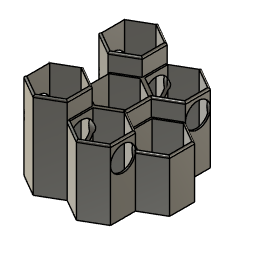
hexagone_rangement v3 (Autodesk Fusion 360 design; units mm, degrees)
Autodesk Fusion 360 part; units mm, degrees
sketch "Esquisse1" plane through (0, 0, 0) normal (0, 0, 1) x (1, 0, 0)
  line L0 (12.5, 7.2169) -> (0, 14.4338)
  line L1 (0, 14.4338) -> (-12.5, 7.2169)
  line L2 (-12.5, 7.2169) -> (-12.5, -7.2169)
  line L3 (-12.5, -7.2169) -> (0, -14.4338)
  line L4 (0, -14.4338) -> (12.5, -7.2169)
  line L5 (12.5, -7.2169) -> (12.5, 7.2169)
  line L6 (0, 14.4338) -> (12.5, 7.2169)
  line L7 (12.5, 7.2169) -> (25, 14.4338)
  line L8 (25, 14.4338) -> (25, 28.8675)
  line L9 (25, 28.8675) -> (12.5, 36.0844)
  line L10 (12.5, 36.0844) -> (0, 28.8675)
  line L11 (0, 28.8675) -> (0, 14.4338)
  line L12 (0, 28.8675) -> (12.5, 36.0844)
  line L13 (12.5, 36.0844) -> (12.5, 50.5181)
  line L14 (12.5, 50.5181) -> (0, 57.735)
  line L15 (0, 57.735) -> (-12.5, 50.5181)
  line L16 (-12.5, 50.5181) -> (-12.5, 36.0844)
  line L17 (-12.5, 36.0844) -> (0, 28.8675)
  line L18 (12.5, 7.2169) -> (12.5, -7.2169)
  line L19 (12.5, -7.2169) -> (25, -14.4338)
  line L20 (25, -14.4338) -> (37.5, -7.2169)
  line L21 (37.5, -7.2169) -> (37.5, 7.2169)
  line L22 (37.5, 7.2169) -> (25, 14.4338)
  line L23 (25, 14.4338) -> (12.5, 7.2169)
  line L24 (12.5, 36.0844) -> (25, 28.8675)
  line L25 (25, 28.8675) -> (37.5, 36.0844)
  line L26 (37.5, 36.0844) -> (37.5, 50.5181)
  line L27 (37.5, 50.5181) -> (25, 57.735)
  line L28 (25, 57.735) -> (12.5, 50.5181)
  line L29 (12.5, 50.5181) -> (12.5, 36.0844)
  line L30 (25, 28.8675) -> (25, 14.4338)
  line L31 (25, 14.4338) -> (37.5, 7.2169)
  line L32 (37.5, 7.2169) -> (50, 14.4338)
  line L33 (50, 14.4338) -> (50, 28.8675)
  line L34 (50, 28.8675) -> (37.5, 36.0844)
  line L35 (37.5, 36.0844) -> (25, 28.8675)
  line L36 (0, 13.2791) -> (-11.5, 6.6395)
  line L37 (-11.5, 6.6395) -> (-11.5, -6.6395)
  line L38 (-11.5, -6.6395) -> (0, -13.2791)
  line L39 (0, -13.2791) -> (11.5, -6.6395)
  line L40 (11.5, -6.6395) -> (11.5, 6.6395)
  line L41 (0, 13.2791) -> (11.5, 6.6395)
  line L42 (13.5, -6.6395) -> (25, -13.2791)
  line L43 (25, -13.2791) -> (36.5, -6.6395)
  line L44 (36.5, -6.6395) -> (36.5, 6.6395)
  line L45 (36.5, 6.6395) -> (25, 13.2791)
  line L46 (25, 13.2791) -> (13.5, 6.6395)
  line L47 (13.5, -6.6395) -> (13.5, 6.6395)
  line L48 (26, 15.0111) -> (26, 28.2902)
  line L49 (26, 28.2902) -> (37.5, 34.9297)
  line L50 (49, 28.2902) -> (37.5, 34.9297)
  line L51 (49, 15.0111) -> (49, 28.2902)
  line L52 (37.5, 8.3716) -> (49, 15.0111)
  line L53 (37.5, 8.3716) -> (26, 15.0111)
  line L54 (1, 28.2902) -> (12.5, 34.9297)
  line L55 (24, 28.2902) -> (12.5, 34.9297)
  line L56 (24, 28.2902) -> (24, 15.0111)
  line L57 (12.5, 8.3716) -> (24, 15.0111)
  line L58 (12.5, 8.3716) -> (1, 15.0111)
  line L59 (1, 28.2902) -> (1, 15.0111)
  line L60 (13.5, 36.6617) -> (13.5, 49.9408)
  line L61 (25, 56.5803) -> (13.5, 49.9408)
  line L62 (36.5, 49.9408) -> (25, 56.5803)
  line L63 (36.5, 36.6617) -> (36.5, 49.9408)
  line L64 (36.5, 36.6617) -> (25, 30.0222)
  line L65 (25, 30.0222) -> (13.5, 36.6617)
  line L66 (11.5, 36.6617) -> (11.5, 49.9408)
  line L67 (11.5, 49.9408) -> (0, 56.5803)
  line L68 (0, 56.5803) -> (-11.5, 49.9408)
  line L69 (-11.5, 49.9408) -> (-11.5, 36.6617)
  line L70 (-11.5, 36.6617) -> (0, 30.0222)
  line L71 (0, 30.0222) -> (11.5, 36.6617)
  point P0 (12.5, 21.6506)
  point P1 (0, 43.3013)
  point P2 (25, 0)
  point P3 (25, 43.3013)
  point P4 (37.5, 21.6506)
  dimension "d5" = 25
  dimension "d10" = 1
  dimension "d11" = 1
  measures "d5" distance of L2 L5
extrude "Extrusion1" add sketch "Esquisse1" along normal blind 50 contours L0 L1 L2 L3 L4 L5 L6 L18 | L10 L12 L13 L14 L15 L16 L17 L29 makes body 1 at (12.5, -2.4056, 16.6667) makes body 2 at (-4.1667, 55.3294, 16.6667)
extrude "Extrusion2" add sketch "Esquisse1" along normal blind 40 contours L5 L7 L18 L19 L20 L21 L22 L23 L31 | L0 L6 L7 L8 L9 L10 L11 L12 L23 L24 L30 | L9 L13 L24 L25 L26 L27 L28 L29 L35 bodies 1 2
extrude "Extrusion3" add sketch "Esquisse1" along normal blind 30 contours L8 L22 L25 L30 L31 L32 L33 L34 L35 bodies 1
extrude "Extrusion4" add sketch "Esquisse1" along normal blind 2 contours L36 L37 L38 L39 L40 L41 | L42 L43 L44 L45 L46 L47 | L48 L49 L50 L51 L52 L53 | L54 L55 L56 L57 L58 L59 | L60 L61 L62 L63 L64 L65 | L66 L67 L68 L69 L70 L71 bodies 1
sketch "Esquisse3" plane through (37.5, 0, 0) normal (1, 0, 0) x (0, 1, 0)
  line L0 (-7.2169, 0) -> (7.2169, 0)
  line L1 (7.2169, 0) -> (7.2169, 30)
  line L2 (7.2169, 30) -> (7.2169, 40)
  line L3 (7.2169, 40) -> (-7.2169, 40)
  line L4 (-7.2169, 40) -> (-7.2169, 0)
  circle A0 centre (0, 30) radius 7.2169
  constraint coincident L1.end A0
extrude "Extrusion5" cut sketch "Esquisse3" against normal blind 71 contours A0 bodies 1
sketch "Esquisse4" plane through (37.5, 0, 0) normal (1, 0, 0) x (0, 1, 0)
  line L0 (36.0844, 0) -> (50.5181, 0)
  line L1 (50.5181, 0) -> (50.5181, 40)
  line L2 (50.5181, 40) -> (36.0844, 40)
  line L3 (36.0844, 40) -> (36.0844, 30)
  line L4 (36.0844, 30) -> (36.0844, 0)
  circle A0 centre (43.3013, 30) radius 7.2169
extrude "Extrusion6" cut sketch "Esquisse4" against normal blind 55 contours A0 bodies 1
fillet "Congé1" radius 1 3 edges at (43.75, 10.8253, 30) (50, 21.6506, 30) (43.75, 32.476, 30) on bodies 1
fillet "Congé2" radius 1 10 edges at (18.75, -10.8253, 40) (31.25, -10.8253, 40) (37.5, 0, 40) (31.25, 10.8253, 40) (25, 21.6506, 40) (31.25, 32.476, 40) (37.5, 43.3013, 40) (31.25, 54.1266, 40) (18.75, 54.1266, 40) (0, 21.6506, 40) on bodies 1
fillet "Congé3" radius 1 6 edges at (-6.25, -10.8253, 50) (-12.5, 0, 50) (-6.25, 10.8253, 50) (6.25, 10.8253, 50) (12.5, 0, 50) (6.25, -10.8253, 50) on bodies 1
fillet "Congé4" radius 1 6 edges at (-6.25, 32.476, 50) (6.25, 32.476, 50) (12.5, 43.3013, 50) (6.25, 54.1266, 50) (-6.25, 54.1266, 50) (-12.5, 43.3013, 50) on bodies 1
equation "largeur_hexa = 25 mm"
equation "hauteur_1 = 30 mm"
equation "hauteur_2 = 40 mm"
equation "hauteur_3 = 50 mm"
equation "d5 = largeur_hexa"
equation "largeur_paroi = 1 mm"
equation "d9 = -largeur_paroi"
equation "d10 = largeur_paroi"
equation "d11 = largeur_paroi"
equation "d12 = -largeur_paroi"
equation "d13 = -largeur_paroi"
equation "d14 = -largeur_paroi"
equation "d15 = hauteur_3"
equation "d17 = hauteur_2"
equation "d19 = hauteur_1"
equation "hauteur_base = 2 mm"
equation "d22 = hauteur_base"
